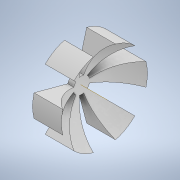
# Autodesk Inventor part: 2020plateForBall
Saved by Autodesk Inventor 2022.2 (Build 262287000, 287)
## iProperties
Created: 2020-01-14
Part Number: 2020plateForBall
Material: Generic
Document SubType Name: Modeling
Designer: steele
Density: 1 g/cm^3
Appearance: Default
Author: steele
Autodesk Inventor part; units mm, degrees
ref_plane "YZ Plane" through (0, 0, 0) normal (1, 0, 0) x (0, 1, 0)
ref_plane "XZ Plane" through (0, 0, 0) normal (0, 1, 0) x (-1, 0, 0)
ref_plane "XY Plane" through (0, 0, 0) normal (0, 0, 1) x (1, 0, 0)
sketch "Sketch4" plane through (0, 0, 0) normal (0, 0, 1) x (1, 0, 0)
  line L0 (0, 0) -> (101.6, 0) construction
  arc A0 (68.2819, 101.6) -> (12.7, 0) centre (133.35, 0) ccw
  line L1 (12.7, 0) -> (12.7, 96.7762) construction
  line L2 (0, 0) -> (0, 101.6)
  line L3 (0, 101.6) -> (68.2819, 101.6)
  line L4 (0, 0) -> (12.7, 0)
  dimension "d11" = 101.6
  dimension "d12" = 12.7
  dimension "d13" = 101.6
  dimension "d14" = 241.3
  constraints: 10 end point, 2 point on circle, 2 point on line, 2 vertical, 1 centre point, 1 collinear, 1 horizontal, 1 perpendicular, 1 tangent
  measures "d11" distance of L0.start L0.end
  measures "d12" distance from line of L0.start L1
  measures "d13" distance of L0.start L2.end
  measures "d14" diameter of A0
revolve "Revolution2" add sketch "Sketch4" angle 360 about axis through (0, 0, 0) along (1, 0, 0)
sketch "Sketch5" plane through (0, 0, 0) normal (-1, 0, 0) x (0, 0, 1)
  arc A0 (4.9305, 18.4009) -> (-4.9305, 18.4009) centre (0, 0) ccw
  circle A1 centre (0, 0) radius 101.6 projected
  arc A2 (26.296, 98.1381) -> (-26.296, 98.1381) centre (0, 0) ccw
  line L0 (-4.9305, 18.4009) -> (-26.296, 98.1381)
  circle A3 centre (0, 0) radius 101.6 projected
  line L1 (0, 0) -> (0, 101.6) construction
  line L2 (4.9305, 18.4009) -> (26.296, 98.1381)
  point P0 (26.296, 98.1381)
  point P1 (-26.296, 98.1381)
  dimension "d18" = 38.1
  dimension "d19" = 15
  dimension "d20" = 15
  constraints: 7 point on circle, 6 end point, 2 centre point, 2 coincident, 1 vertical
  measures "d18" diameter of A0
  measures "d19" angle of L0 L1
  measures "d20" angle of L1 L2
extrude "Extrusion4" cut sketch "Sketch5" against normal through all contours A0 L0 A1 L2 picked at (-14.8293, 72.4233)
pattern_circular "Circular Pattern1" count 6 over 360 about axis through (-10, 0, 0) along (1, 0, 0) of "Extrusion4"
body "Solid3"
